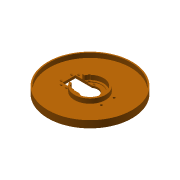
# Autodesk Inventor part: P_ankle01_001
Saved by Autodesk Inventor 2016 (Build 200138000, 138)
## iProperties
Created: 2016-02-23
Part Number: P_ankle01_001
Material: PC/ABS Plastic
Document SubType Name: Modeling
Designer: Mateusz
Density: 0.357273 g/cm^3
Appearance: Orange
Author: Mateusz
Autodesk Inventor part; units mm, degrees
ref_plane "YZ Plane" through (0, 0, 0) normal (1, 0, 0) x (0, 1, 0)
ref_plane "XZ Plane" through (0, 0, 0) normal (0, 1, 0) x (-1, 0, 0)
ref_plane "XY Plane" through (0, 0, 0) normal (0, 0, 1) x (1, 0, 0)
derived "skeleton.ipt"
sketch "Sketch1" plane through (0, 0, 0) normal (0, 0, 1) x (1, 0, 0)
  line L0 (-91, 0) -> (91, 0) projected
  line L1 (0, 91) -> (0, -91) projected
  line L2 (15, 19) -> (-43, 19)
  line L3 (-43, 19) -> (-43, -19)
  line L4 (-43, -19) -> (15, -19)
  line L5 (15, -19) -> (15, 19)
  circle A0 centre (0, 0) radius 3.1 projected
  circle A1 centre (-8, 0) radius 1.25 projected
  circle A2 centre (0, -8) radius 1.25 projected
  circle A3 centre (8, 0) radius 1.25 projected
  circle A4 centre (0, -5.5) radius 0.75 projected
  circle A5 centre (-4.7631, 2.75) radius 0.75 projected
  circle A6 centre (4.7631, 2.75) radius 0.75 projected
  arc A7 (-0.2472, 9.2253) -> (0.2472, 9.2253) centre (0, 8) ccw projected
  line L6 (-0.2472, 9.2253) -> (-0.2472, 10.9972) projected
  arc A8 (-0.2472, 10.9972) -> (-1.15, -10.9397) centre (0, 0) ccw projected
  line L7 (-1.15, -10.9397) -> (-1.15, -10.6) projected
  line L8 (-1.15, -10.6) -> (-0.85, -10.6) projected
  line L9 (-0.85, -10.6) -> (-0.85, -10.9671) projected
  arc A9 (-0.85, -10.9671) -> (0.85, -10.9671) centre (0, 0) ccw projected
  line L10 (0.85, -10.9671) -> (0.85, -10.6) projected
  line L11 (0.85, -10.6) -> (1.15, -10.6) projected
  line L12 (1.15, -10.6) -> (1.15, -10.9397) projected
  arc A10 (1.15, -10.9397) -> (0.2472, 10.9972) centre (0, 0) ccw projected
  line L13 (0.2472, 10.9972) -> (0.2472, 9.2253) projected
  circle A11 centre (-6.5, 13.5) radius 1.1 projected
  circle A12 centre (-14.5, 13.5) radius 1.1 projected
  circle A13 centre (-22.5, 13.5) radius 1.1 projected
  circle A14 centre (-30.5, 13.5) radius 1.1 projected
  circle A15 centre (-36, 8) radius 1.1 projected
  circle A16 centre (-36, -8) radius 1.1 projected
  circle A17 centre (-30.5, -13.5) radius 1.1 projected
  circle A18 centre (-22.5, -13.5) radius 1.1 projected
  circle A19 centre (-14.5, -13.5) radius 1.1 projected
  circle A20 centre (-6.5, -13.5) radius 1.1 projected
  line L14 (-3.2, 16) -> (-9.8, 16) projected
  line L15 (-9.8, -16) -> (-3.2, -16) projected
  line L16 (-38.5, -4.7) -> (-38.5, -11.3) projected
  line L17 (-38.5, 11.3) -> (-38.5, 4.7) projected
  line L18 (11.5, 7) -> (11.5, 0.1) projected
  line L19 (11.5, -0.1) -> (11.5, -7) projected
  line L20 (-32.5, -8.3063) -> (-32.5, 8.3063) projected
  line L21 (-8.8, 9.2) -> (-30.8063, 9.2) projected
  line L22 (-8.8, -10) -> (-30.8063, -10) projected
  arc A21 (2.6308, -11.7081) -> (-1.8888, 11.8504) centre (0, 0) ccw
  arc A22 (0.7846, -11.9743) -> (2.6308, -11.7081) centre (0, 0) ccw
  arc A23 (-1.8888, 11.8504) -> (0.7846, -11.9743) centre (0, 0) ccw
  line L23 (12.0079, 7) -> (12.0079, 0.1)
  circle A24 centre (0, 0) radius 60
  point P0 (0, 0)
  dimension "d0" = 1
  dimension "d1" = 58
  dimension "d2" = 38
  dimension "d3" = 15
  dimension "d28" = 120
  constraints: 10 end point, 6 point on circle, 4 centre point, 3 parallel, 1 coincident, 1 horizontal, 1 perpendicular, 3 other
  measures "d0" radial gap between concentric circles of A10 A21
  measures "d1" distance between parallel lines of L5 L3
  measures "d2" distance between parallel lines of L2 L4
  measures "d3" distance between parallel lines of L5 L1
  measures "d28" diameter of A24
extrude "Extrusion1" add sketch "Sketch1" along normal blind 4 contours A24 L1 L2 L3 L0 | L0 L3 L4 L1 A24 | L3 L2 L1 A21 A23 L0 | L0 A23 L1 L4 L3 | A24 L0 L5 L2 L1 | L1 L4 L5 L0 A24 | L2 L5 L0 A21 L1 | L1 A23 A22 A21 L0 L5 L4 | A11 | A12 | A13 | A14 | A15 | A16 | A17 | A18 | A19 | A20
sketch "Sketch2" plane through (0, 0, 0) normal (0, 0, -1) x (-1, 0, 0)
  line L0 (8.8, -10) -> (30.8063, -10) projected
  line L1 (30.8063, 10) -> (8.8, 10) projected
  line L2 (37, -4.7) -> (37, 4.7) projected
  line L3 (32.5, -8.3063) -> (32.5, 8.3063) projected
  circle A0 centre (0, 0) radius 12 projected
  line L4 (32.5, 10) -> (6.6332, 10)
  line L5 (6.6332, 10) -> (6.6332, -10)
  line L6 (6.6332, -10) -> (32.5, -10)
  line L7 (32.5, -10) -> (32.5, 10)
  point P0 (0, 0)
  constraints: 8 end point, 3 collinear, 2 parallel, 1 horizontal, 1 perpendicular, 2 other
extrude "Extrusion2" cut sketch "Sketch2" against normal up to next contours L6 A0 L4 L1 L7 L3 L0 | L5 A0 picked at (8.6926, -2.5312)
sketch "Sketch3" plane through (0, 0, 0) normal (0, 0, -1) x (-1, 0, 0)
  circle A0 centre (6.5, 13.5) radius 1.1 projected
  circle A1 centre (14.5, 13.5) radius 1.1 projected
  circle A2 centre (22.5, 13.5) radius 1.1 projected
  circle A3 centre (30.5, 13.5) radius 1.1 projected
  circle A4 centre (36, 8) radius 1.1 projected
  circle A5 centre (36, -8) radius 1.1 projected
  circle A6 centre (30.5, -13.5) radius 1.1 projected
  circle A7 centre (22.5, -13.5) radius 1.1 projected
  circle A8 centre (14.5, -13.5) radius 1.1 projected
  circle A9 centre (6.5, -13.5) radius 1.1 projected
  point P0 (0, 0)
  constraints: 10 coincident
hole "Hole1" at (-6.5, -13.5, 0) at (-14.5, -13.5, 0) at (-22.5, -13.5, 0) at (-30.5, -13.5, 0) at (-36, -8, 0) at (-36, 8, 0) at (-30.5, 13.5, 0) at (-22.5, 13.5, 0) at (-14.5, 13.5, 0) at (-6.5, 13.5, 0) direction (0, 0, 1) diameter 2.2 end through all
sketch "Sketch7" plane through (0, 0, 4) normal (0, 0, 1) x (1, 0, 0)
  circle A0 centre (0, 0) radius 60 projected
  circle A1 centre (0, 0) radius 18
  point P0 (0, 0)
  dimension "d29" = 36
  constraints: 1 centre point, 1 coincident
  measures "d29" diameter of A1
extrude "Extrusion6" cut sketch "Sketch7" against normal blind 1 contours A1
chamfer "Chamfer1" distance 1 angle 45 10 edges at (-30.5, -14.6, 4) (-36, -9.1, 4) (-36, 6.9, 4) (-30.5, 12.4, 4) (-22.5, 12.4, 4) (-14.5, 12.4, 4) (-6.5, 12.4, 3) (-22.5, -14.6, 4) (-14.5, -14.6, 4) (-6.5, -14.6, 3)
sketch "Sketch8" plane through (0, 0, 4) normal (0, 0, 1) x (1, 0, 0)
  circle A0 centre (0, 0) radius 60 projected
  arc A1 (-14.9666, -10) -> (-14.9666, 10) centre (0, 0) ccw projected
  arc A2 (-21.8174, -10) -> (-21.8174, 10) centre (0, 0) ccw
  arc A3 (-13.8428, -11.5055) -> (-12.4637, -12.9868) centre (-14.5, -13.5) ccw projected
  arc A4 (-12.4637, 12.9868) -> (-13.8428, 11.5055) centre (-14.5, 13.5) ccw projected
  line L0 (-14.9666, -10) -> (-32.5, -10) projected
  line L1 (-32.5, 10) -> (-14.9666, 10) projected
  arc A5 (-18.4662, -10) -> (-16.528, -12.9548) centre (0, 0) ccw
  arc A6 (-14.1008, -15.5617) -> (-14.1008, 15.5617) centre (0, 0) ccw
  arc A7 (-16.528, 12.9548) -> (-18.4662, 10) centre (0, 0) ccw
  point P0 (0, 0)
  dimension "d37" = 24
  dimension "d38" = 21
  dimension "d39" = 21
  dimension "d40" = 21
  constraints: 12 point on circle, 4 centre point, 4 point on line, 1 coincident
  measures "d37" radius of A2
  measures "d38" radius of A6
  measures "d39" radius of A7
  measures "d40" radius of A5
extrude "Extrusion7" add sketch "Sketch8" along normal blind 7 contours A5 A3 A6 A4 A7 L1 A2 L0
sketch "Sketch9" plane through (0, 0, 4) normal (0, 0, 1) x (1, 0, 0)
  circle A0 centre (0, 0) radius 60 projected
  circle A1 centre (0, 0) radius 58
  point P0 (0, 0)
  dimension "d43" = 2
  constraints: 1 centre point
  measures "d43" radial gap between concentric circles of A0 A1
extrude "Extrusion8" add sketch "Sketch9" along normal blind 7
sketch "Sketch10" plane through (0, 0, 4) normal (0, 0, 1) x (1, 0, 0)
  circle A0 centre (27.57, -9.8473) radius 1.65 projected
  circle A1 centre (27.57, 9.8473) radius 1.65 projected
  point P0 (0, 0)
extrude "Extrusion9" cut sketch "Sketch10" against normal through all
body "Solid1"
